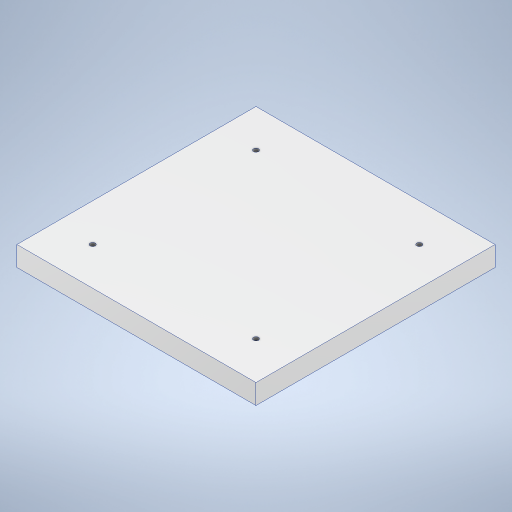
# Autodesk Inventor part: BasePlate
Saved by Autodesk Inventor 2023 (Build 270158000, 158)
## iProperties
Created: 2023-09-26
Part Number: BasePlate
Material: Aluminum 6061
Document SubType Name: Modeling
Designer: Gage
Density: 2.7 g/cm^3
Appearance: Aluminum - Flat
Author: Gage
Autodesk Inventor part; units mm, degrees
ref_plane "YZ Plane" through (0, 0, 0) normal (1, 0, 0) x (0, 1, 0)
ref_plane "XZ Plane" through (0, 0, 0) normal (0, 1, 0) x (-1, 0, 0)
ref_plane "XY Plane" through (0, 0, 0) normal (0, 0, 1) x (1, 0, 0)
sketch "Sketch1" plane through (0, 0, 0) normal (0, 1, 0) x (-1, 0, 0)
  line L0 (76.2, -76.2) -> (-76.2, -76.2)
  line L1 (-76.2, -76.2) -> (-76.2, 76.2)
  line L2 (-76.2, 76.2) -> (76.2, 76.2)
  line L3 (76.2, 76.2) -> (76.2, -76.2)
  point P0 (0, 0)
  point P1 (-76.2, 0)
  point P2 (0, -76.2)
  dimension "d0" = 152.4
  dimension "d1" = 152.4
  constraints: 8 end point, 2 midpoint, 2 parallel, 1 horizontal, 1 horizontal alignment, 1 perpendicular, 1 vertical alignment
  measures "d0" distance of L1.end L2.end
  measures "d1" distance of L0.end L1.end
extrude "Extrusion1" add sketch "Sketch1" along normal blind 12.7
sketch "Sketch3" plane through (0, 12.7, 0) normal (0, 1, 0) x (1, 0, 0)
  line L0 (-57.15, 57.15) -> (57.15, 57.15)
  line L1 (57.15, 57.15) -> (57.15, -57.15)
  line L2 (57.15, -57.15) -> (-57.15, -57.15)
  line L3 (-57.15, -57.15) -> (-57.15, 57.15)
  point P0 (0, 0)
  point P1 (-57.15, 0)
  point P2 (0, 57.15)
  point P3 (-52.07, 52.07)
  point P4 (52.07, 52.07)
  point P5 (52.07, -52.07)
  point P6 (-52.07, -52.07)
  dimension "d17" = 114.3
  dimension "d18" = 114.3
  dimension "d26" = 5.08
  dimension "d27" = 5.08
  dimension "d28" = 5.08
  dimension "d29" = 5.08
  dimension "d30" = 5.08
  dimension "d31" = 5.08
  dimension "d32" = 5.08
  dimension "d33" = 5.08
  constraints: 8 end point, 2 midpoint, 2 parallel, 1 horizontal, 1 horizontal alignment, 1 perpendicular, 1 vertical alignment
  measures "d17" distance of L1.end L2.end
  measures "d18" distance of L0.end L1.end
  measures "d26" distance from line of L0 point (-52.07, 52.07)
  measures "d27" distance from line of point (-52.07, 52.07) L3
  measures "d28" distance from line of L2 point (52.07, -52.07)
  measures "d29" distance from line of L1 point (52.07, -52.07)
  measures "d30" distance from line of L2 point (-52.07, -52.07)
  measures "d31" distance from line of L3 point (-52.07, -52.07)
  measures "d32" distance from line of L1 point (52.07, 52.07)
  measures "d33" distance from line of point (52.07, 52.07) L0
hole "Hole1" at (-52.07, 12.7, -52.07) at (52.07, 12.7, -52.07) at (52.07, 12.7, 52.07) at (-52.07, 12.7, 52.07) direction (0, -1, 0) diameter 3.302 end through all thread size "8-32 UNC" class "2B" standard "ANSI Unified Screw Threads"
sketch "Sketch4" plane through (0, 12.7, 0) normal (0, 1, 0) x (1, 0, 0)
  line L0 (-55.5625, 55.4863) -> (58.7375, 55.4863)
  line L1 (58.7375, 55.4863) -> (58.7375, -58.8137)
  line L2 (58.7375, -58.8137) -> (-55.5625, -58.8137)
  line L3 (-55.5625, -58.8137) -> (-55.5625, 55.4863)
  line L4 (-30.1625, -52.4129) -> (23.1775, -52.4129)
  line L5 (23.1775, -52.4129) -> (23.1775, 49.1871)
  line L6 (23.1775, 49.1871) -> (-30.1625, 49.1871)
  line L7 (-30.1625, 49.1871) -> (-30.1625, -52.4129)
  circle A0 centre (-27.6225, -37.1729) radius 1.5875
  circle A1 centre (20.6375, -38.4429) radius 1.5875
  circle A2 centre (20.6375, 44.1071) radius 1.5875
  circle A3 centre (-27.6225, 37.7571) radius 1.5875
  point P0 (0, 0)
  dimension "d34" = 114.3
  dimension "d35" = 114.3
  dimension "d36" = 53.34
  dimension "d37" = 101.6
  dimension "d38" = 3.175
  dimension "d39" = 15.24
  dimension "d40" = 2.54
  dimension "d41" = 2.54
  dimension "d42" = 13.97
  dimension "d43" = 96.52
  dimension "d44" = 2.54
  dimension "d45" = 90.17
  dimension "d46" = 2.54
  dimension "d47" = 25.4
  dimension "d70" = 6.4008
  constraints: 16 end point, 4 centre point, 4 parallel, 2 horizontal, 2 perpendicular
  measures "d34" distance of L1.end L2.end
  measures "d35" distance of L0.end L1.end
  measures "d36" distance of L6.end L5.end
  measures "d37" distance of L5.end L4.end
  measures "d38" diameter of A0
  measures "d39" distance from line of L4 A0.centre
  measures "d40" distance from line of L7 A0.centre
  measures "d41" distance from line of L5 A1.centre
  measures "d42" distance from line of L4 A1.centre
  measures "d43" distance from line of L4 A2.centre
  measures "d44" distance from line of L5 A2.centre
  measures "d45" distance from line of L4 A3.centre
  measures "d46" distance from line of L7 A3.centre
  measures "d47" distance between parallel lines of L7 L3
  measures "d70" distance between parallel lines of L2 L4
hole "Hole2" [suppressed]
sketch "Sketch7" plane through (0, 0, 0) normal (0, -1, 0) x (1, 0, 0)
  circle A0 centre (-27.6225, 37.1729) radius 3.3782 projected
  circle A1 centre (-27.6225, 37.1729) radius 6.35
  circle A2 centre (20.6375, 38.4429) radius 3.3782 projected
  circle A3 centre (20.6375, 38.4429) radius 6.35
  circle A4 centre (20.6375, -44.1071) radius 3.3782 projected
  circle A5 centre (20.6375, -44.1071) radius 6.35
  circle A6 centre (-27.6225, -37.7571) radius 3.3782 projected
  circle A7 centre (-27.6225, -37.7571) radius 6.35
  point P0 (0, 0)
  dimension "d63" = 12.7
  dimension "d64" = 12.7
  dimension "d65" = 12.7
  dimension "d66" = 12.7
  constraints: 4 centre point, 4 coincident
  measures "d63" diameter of A1
  measures "d64" diameter of A3
  measures "d65" diameter of A5
  measures "d66" diameter of A7
extrude "Extrusion3" [suppressed]
body "Solid1"
